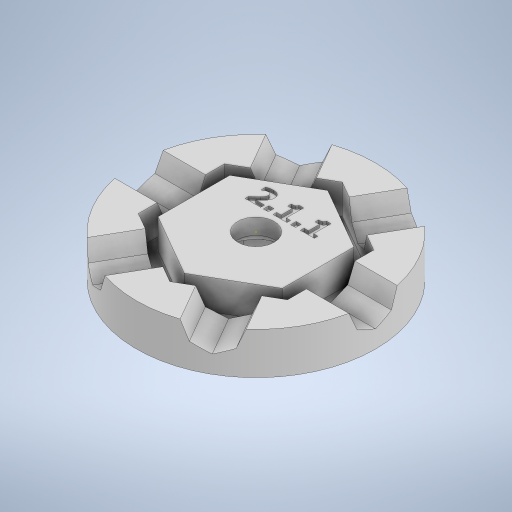
# Autodesk Inventor part: WindHub
Saved by Autodesk Inventor 2024.3 (Build 283343000, 343)
## iProperties
Created: 2024-11-22
Part Number: WindHub
Material: Generisch
Document SubType Name: Modeling
Designer: Maximilian Hock
Density: 1 g/cm^3
Appearance: Vorgabe
Author: Maximilian Hock
## iProperties of the stored document MemberDocs/x13ze2sctPcs3c0rvDhmze2odJh
Created: 2024-11-22
Part Number: WindHub
Material: Generisch
Document SubType Name: Modeling
Designer: Maximilian Hock
Density: 1 g/cm^3
Appearance: Vorgabe
Author: Maximilian Hock
## iProperties of the stored document WindHub_3D-Druck.ipt
Created: 2025-02-12
Part Number: WindHub_3D-Druck
Material: Generisch
Document SubType Name: Modeling
Designer: Maximilian Hock
Density: 1 g/cm^3
Appearance: Vorgabe
Author: Maximilian Hock
Autodesk Inventor part; units mm, degrees
ref_plane "YZ Plane" through (0, 0, 0) normal (1, 0, 0) x (0, 1, 0)
ref_plane "XZ Plane" through (0, 0, 0) normal (0, 1, 0) x (-1, 0, 0)
ref_plane "XY Plane" through (0, 0, 0) normal (0, 0, 1) x (1, 0, 0)
sketch "Skizze1" plane through (0, 0, 0) normal (0, 0, 1) x (1, 0, 0)
  circle A0 centre (0, 0) radius 20
  dimension "d0" = 40
  constraints: 1 centre point, 1 coincident
  measures "d0" diameter of A0
extrude "Extrusion1" add sketch "Skizze1" along normal blind 7
sketch "Skizze3" plane through (0, 0, 7) normal (0, 0, 1) x (1, 0, 0)
  line L0 (0, 12) -> (10.3923, 6)
  line L1 (10.3923, 6) -> (10.3923, -6)
  line L2 (10.3923, -6) -> (0, -12)
  line L3 (0, -12) -> (-10.3923, -6)
  line L4 (-10.3923, -6) -> (-10.3923, 6)
  line L5 (-10.3923, 6) -> (0, 12)
  line L6 (0, 14.4249) -> (12.4923, 7.2124)
  line L7 (12.4923, 7.2124) -> (12.4923, -7.2124)
  line L8 (12.4923, -7.2124) -> (0, -14.4249)
  line L9 (0, -14.4249) -> (-12.4923, -7.2124)
  line L10 (-12.4923, -7.2124) -> (-12.4923, 7.2124)
  line L11 (-12.4923, 7.2124) -> (0, 14.4249)
  point P0 (0, 0)
  point P1 (0, 0)
  dimension "d6" = 12
  dimension "d7" = 2.1
  constraints: 24 end point, 1 coincident, 1 vertical alignment, 18 other
  measures "d6" distance of L0.start L0.end
  measures "d7" distance between parallel lines of L11 L5
extrude "Extrusion2" cut sketch "Skizze3" against normal blind 5
sketch "Skizze2" plane through (10.3923, 0, -13) normal (1, 0, 0) x (0, 1, 0)
  line L0 (0, 25.05) -> (3.5709, 23.5709)
  line L1 (3.5709, 23.5709) -> (5.05, 20)
  line L2 (5.05, 20) -> (3.5709, 16.4291)
  line L3 (3.5709, 16.4291) -> (0, 14.95)
  line L4 (0, 14.95) -> (-3.5709, 16.4291)
  line L5 (-3.5709, 16.4291) -> (-5.05, 20)
  line L6 (-5.05, 20) -> (-3.5709, 23.5709)
  line L7 (-3.5709, 23.5709) -> (0, 25.05)
  line L8 (0, 24.05) -> (2.8638, 22.8638)
  line L9 (2.8638, 22.8638) -> (4.05, 20)
  line L10 (4.05, 20) -> (2.8638, 17.1362)
  line L11 (2.8638, 17.1362) -> (0, 15.95)
  line L12 (0, 15.95) -> (-2.8638, 17.1362)
  line L13 (-2.8638, 17.1362) -> (-4.05, 20)
  line L14 (-4.05, 20) -> (-2.8638, 22.8638)
  line L15 (-2.8638, 22.8638) -> (0, 24.05)
  line L16 (6, 20) -> (-6, 20) projected
  point P0 (0, 13)
  point P1 (0, 20)
  dimension "d3" = 10.1
  dimension "d11" = 8.1
  constraints: 32 end point, 2 vertical alignment, 1 midpoint, 24 other
  measures "d3" distance of L3.end L0.start
  measures "d11" distance of L11.end L8.start
extrude "Extrusion3" cut sketch "Skizze2" along normal through all contours L16 L14 L15 L8 L9 | L10 L11 L12 L13 L16
pattern_circular "Runde Anordnung1" count 6 over 360 about axis through (0, 0, 0) along (0, 0, 1) of "Extrusion3"
sketch "Skizze7" plane through (0, 0, 0) normal (0, 0, -1) x (-1, 0, 0)
  point P0 (0, 0)
  point P1 (0, 0)
  constraints: 1 coincident
hole "Bohrung3" at (0, 0, 0) direction (0, 0, 1) diameter 6.1 end through all
sketch "Skizze8" plane through (0, 0, 0) normal (0, 0, -1) x (-1, 0, 0)
  line L0 (0, 5.8235) -> (5.0433, 2.9117)
  line L1 (5.0433, 2.9117) -> (5.0433, -2.9118)
  line L2 (5.0433, -2.9118) -> (0, -5.8235)
  line L3 (0, -5.8235) -> (-5.0433, -2.9118)
  line L4 (-5.0433, -2.9118) -> (-5.0433, 2.9118)
  line L5 (-5.0433, 2.9118) -> (0, 5.8235)
  point P0 (0, 0)
  point P1 (0, 0)
  dimension "d42" = 11.647
  constraints: 12 end point, 1 coincident, 1 vertical alignment, 13 other
  measures "d42" distance of L2.end L0.start
extrude "Extrusion5" cut sketch "Skizze8" against normal blind 2.35
chamfer "Fasen1" distance 2 angle 45 1 edges at (0, -3.05, 2.35)
sketch "Skizze9" plane through (0, 0, 7) normal (0, 0, 1) x (1, 0, 0)
  point P0 (0, 0)
sketch "Skizze10" plane through (0, 0, 7) normal (0, 0, 1) x (1, 0, 0)
  line L0 (-6.253, 8.3898) -> (6.253, 8.3898) construction
  line L1 (6.253, 8.3898) -> (6.253, 3.05) construction
  line L2 (6.253, 3.05) -> (-6.253, 3.05) construction
  line L3 (-6.253, 3.05) -> (-6.253, 8.3898) construction
  circle A0 centre (0, 0) radius 3.05 projected
  line L4 (0, 12) -> (-10.3923, 6) projected
  line L5 (10.3923, 6) -> (0, 12) projected
  line L6 (-3.1752, 3.9359) -> (-5.7478, 3.9359)
  line L7 (-5.7478, 3.9359) -> (-5.7478, 4.506)
  spline S0 degree 2 poles (-5.7478, 4.506) (-5.4216, 4.7669) (-4.8997, 5.2264) (-4.704, 5.4335) knots 0 0 0 1 2 2 2
  spline S1 degree 2 poles (-4.704, 5.4335) (-4.4459, 5.7029) (-4.2162, 6.1142) (-4.2162, 6.3297) knots 0 0 0 1 2 2 2
  spline S2 degree 2 poles (-4.2162, 6.3297) (-4.2162, 6.5736) (-4.5083, 6.8346) (-4.7692, 6.8346) knots 0 0 0 1 2 2 2
  spline S3 degree 2 poles (-4.7692, 6.8346) (-4.9026, 6.8346) (-5.1408, 6.7694) (-5.2628, 6.7183) knots 0 0 0 1 2 2 2
  spline S4 degree 2 poles (-5.2628, 6.7183) (-5.3819, 6.6644) (-5.5521, 6.551) (-5.5946, 6.5226) knots 0 0 0 1 2 2 2
  line L8 (-5.5946, 6.5226) -> (-5.6627, 6.5226)
  line L9 (-5.6627, 6.5226) -> (-5.6627, 7.2856)
  spline S5 degree 2 poles (-5.6627, 7.2856) (-5.5152, 7.3565) (-4.8855, 7.504) (-4.5934, 7.504) knots 0 0 0 1 2 2 2
  spline S6 degree 2 poles (-4.5934, 7.504) (-3.9694, 7.504) (-3.3284, 6.948) (-3.3284, 6.446) knots 0 0 0 1 2 2 2
  spline S7 degree 2 poles (-3.3284, 6.446) (-3.3284, 6.1369) (-3.6205, 5.5412) (-3.9581, 5.2009) knots 0 0 0 1 2 2 2
  spline S8 degree 2 poles (-3.9581, 5.2009) (-4.1708, 4.991) (-4.5707, 4.6648) (-4.6586, 4.5967) knots 0 0 0 1 2 2 2
  line L10 (-4.6586, 4.5967) -> (-3.1752, 4.5967)
  line L11 (-3.1752, 4.5967) -> (-3.1752, 3.9359)
  line L12 (-1.8705, 3.9359) -> (-2.7016, 3.9359)
  line L13 (-2.7016, 3.9359) -> (-2.7016, 4.8605)
  line L14 (-2.7016, 4.8605) -> (-1.8705, 4.8605)
  line L15 (-1.8705, 4.8605) -> (-1.8705, 3.9359)
  line L16 (1.238, 3.9359) -> (-1.0735, 3.9359)
  line L17 (-1.0735, 3.9359) -> (-1.0735, 4.5457)
  line L18 (-1.0735, 4.5457) -> (-0.3361, 4.5457)
  line L19 (-0.3361, 4.5457) -> (-0.3361, 6.3978)
  line L20 (-0.3361, 6.3978) -> (-1.0735, 6.3978)
  line L21 (-1.0735, 6.3978) -> (-1.0735, 6.9679)
  spline S9 degree 2 poles (-1.0735, 6.9679) (-0.9119, 6.9679) (-0.5914, 7.0104) (-0.4949, 7.0558) knots 0 0 0 1 2 2 2
  spline S10 degree 2 poles (-0.4949, 7.0558) (-0.3843, 7.1125) (-0.2595, 7.3026) (-0.2482, 7.4444) knots 0 0 0 1 2 2 2
  line L22 (-0.2482, 7.4444) -> (0.5176, 7.4444)
  line L23 (0.5176, 7.4444) -> (0.5176, 4.5457)
  line L24 (0.5176, 4.5457) -> (1.238, 4.5457)
  line L25 (1.238, 4.5457) -> (1.238, 3.9359)
  line L26 (2.6987, 3.9359) -> (1.8677, 3.9359)
  line L27 (1.8677, 3.9359) -> (1.8677, 4.8605)
  line L28 (1.8677, 4.8605) -> (2.6987, 4.8605)
  line L29 (2.6987, 4.8605) -> (2.6987, 3.9359)
  line L30 (5.8073, 3.9359) -> (3.4957, 3.9359)
  line L31 (3.4957, 3.9359) -> (3.4957, 4.5457)
  line L32 (3.4957, 4.5457) -> (4.2332, 4.5457)
  line L33 (4.2332, 4.5457) -> (4.2332, 6.3978)
  line L34 (4.2332, 6.3978) -> (3.4957, 6.3978)
  line L35 (3.4957, 6.3978) -> (3.4957, 6.9679)
  spline S11 degree 2 poles (3.4957, 6.9679) (3.6574, 6.9679) (3.9779, 7.0104) (4.0744, 7.0558) knots 0 0 0 1 2 2 2
  spline S12 degree 2 poles (4.0744, 7.0558) (4.185, 7.1125) (4.3098, 7.3026) (4.3211, 7.4444) knots 0 0 0 1 2 2 2
  line L36 (4.3211, 7.4444) -> (5.0869, 7.4444)
  line L37 (5.0869, 7.4444) -> (5.0869, 4.5457)
  line L38 (5.0869, 4.5457) -> (5.8073, 4.5457)
  line L39 (5.8073, 4.5457) -> (5.8073, 3.9359)
  point P0 (0, 3.05)
  constraints: 2 point on line, 1 horizontal, 1 midpoint, 1 vertical alignment, 3 other
emboss "Prägen1" sketch "Skizze10" operation cut depth 0.5 direction (0, 0, -1) contours L6 L7 S0 S1 S2 S3 S4 L8 L9 S5 S6 S7 S8 L10 L11 | L12 L13 L14 L15 | L16 L17 L18 L19 L20 L21 S9 S10 L22 L23 L24 L25 | L26 L27 L28 L29 | L30 L31 L32 L33 L34 L35 S11 S12 L36 L37 L38 L39
equation "\"d0\" = WindHubDiameter"
equation "\"d7\" = WindBladeFootThickness + Clearance"
equation "\"d8\" = 0.5 * WindBladeFootOuterDiameter"
equation "\"d3\" = WindBladeFootOuterDiameter + Clearance"
equation "\"d11\" = WindBladeStemOuterDiameter + Clearance"
equation "\"d35\" = AxleDiameter + Clearance"
equation "\"d42\" = HexnutOuterSize + Clearance"
equation "\"d43\" = 0.5 * HexnutHeight"
equation "\"WindHubDiameter\" = 40"
equation "\"WindBladeFootThickness\" = 2"
equation "\"Clearance\" = 0.1"
equation "\"WindBladeFootOuterDiameter\" = 10"
equation "\"WindBladeStemOuterDiameter\" = 8"
equation "\"AxleDiameter\" = 6"
equation "\"HexnutOuterSize\" = 11.547"
equation "\"HexnutHeight\" = 4.7"
